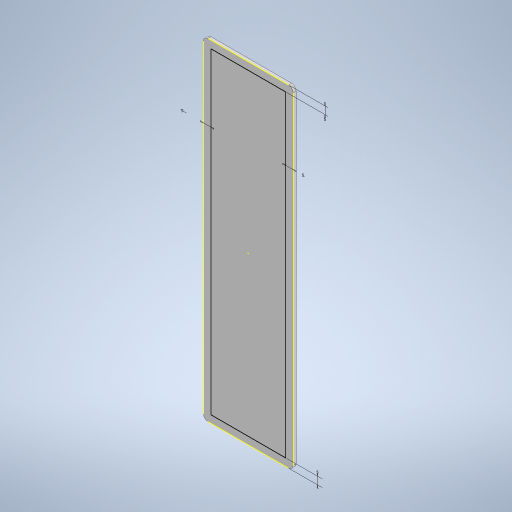
# Autodesk Inventor part: контроль
Saved by Autodesk Inventor 2023.1 (Build 271208000, 208)
## iProperties
Created: 2023-02-15
Part Number: контроль
Material: Типовые
Document SubType Name: Modeling
Designer: User
Density: 1 g/cm^3
Appearance: По умолчанию
Author: User
Autodesk Inventor part; units mm, degrees
ref_plane "YZ Plane" through (0, 0, 0) normal (1, 0, 0) x (0, 1, 0)
ref_plane "XZ Plane" through (0, 0, 0) normal (0, 1, 0) x (-1, 0, 0)
ref_plane "XY Plane" through (0, 0, 0) normal (0, 0, 1) x (1, 0, 0)
sketch "Эскиз1" plane through (0, 0, 0) normal (0, 0, 1) x (1, 0, 0)
  line L0 (-27, 111) -> (27, 111)
  line L1 (30, 108) -> (30, -108)
  line L2 (27, -111) -> (-27, -111)
  line L3 (-30, -108) -> (-30, 108)
  line L4 (0, -156.2698) -> (0, 156.2698) projected
  line L5 (-42.8698, 0) -> (42.8698, 0) projected
  arc A0 (-27, 111) -> (-30, 108) centre (-27, 108) ccw
  arc A1 (30, 108) -> (27, 111) centre (27, 108) ccw
  arc A2 (27, -111) -> (30, -108) centre (27, -108) ccw
  arc A3 (-30, -108) -> (-27, -111) centre (-27, -108) ccw
  point P0 (0, 0)
  dimension "d0" = 60
  dimension "d1" = 222
  dimension "d2" = 3
  constraints: 8 end point, 8 point on circle, 8 tangent, 4 centre point, 3 equal radius, 2 parallel, 1 horizontal, 1 perpendicular, 2 other
  measures "d0" distance between parallel lines of L1 L3
  measures "d1" distance between parallel lines of L2 L0
  measures "d2" radius of A0
extrude "Выдавливание1" add sketch "Эскиз1" along normal blind 2
sketch "Эскиз2" plane through (0, 0, 2) normal (0, 0, 1) x (1, 0, 0)
  line L0 (-25, 106) -> (25, 106)
  line L1 (25, 106) -> (25, -106)
  line L2 (25, -106) -> (-25, -106)
  line L3 (-25, -106) -> (-25, 106)
  line L4 (-30, 108) -> (-30, -108) projected
  line L5 (30, -108) -> (30, 108) projected
  line L6 (27, 111) -> (-27, 111) projected
  line L7 (-27, -111) -> (27, -111) projected
  point P0 (0, 0)
  dimension "d5" = 5
  dimension "d6" = 5
  dimension "d7" = 5
  dimension "d8" = 5
  constraints: 8 end point, 2 parallel, 1 horizontal, 1 perpendicular
  measures "d5" distance between parallel lines of L4 L3
  measures "d6" distance between parallel lines of L5 L1
  measures "d7" distance between parallel lines of L0 L6
  measures "d8" distance between parallel lines of L7 L2
